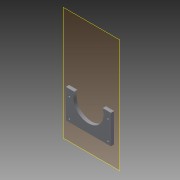
# Autodesk Inventor part: outputGearSupport
Saved by Autodesk Inventor 2013 (Build 170138000, 138)
## iProperties
Created: 2014-07-02
Part Number: outputGearSupport
Material: Generic
Document SubType Name: Modeling
Designer: Nano
Density: 1 g/cm^3
Author: Nano
Autodesk Inventor part; units mm, degrees
ref_plane "YZ Plane" through (0, 0, 0) normal (1, 0, 0) x (0, 1, 0)
ref_plane "XZ Plane" through (0, 0, 0) normal (0, 1, 0) x (-1, 0, 0)
ref_plane "XY Plane" through (0, 0, 0) normal (0, 0, 1) x (1, 0, 0)
ref_plane "Work Plane1" through (0, 0, 0) normal (0, 0, 1) x (1, 0, 0)
sketch "Sketch1" plane through (0, 0, 0) normal (0, 0, 1) x (1, 0, 0)
  circle A0 centre (0, -25.4) radius 24.765 construction
  arc A1 (-28.1777, -15.24) -> (28.1777, -15.24) centre (0, -25.4) ccw
  line L0 (-44.45, -72.39) -> (44.45, -72.39)
  line L1 (44.45, -72.39) -> (44.45, -15.24)
  line L2 (-44.45, -15.24) -> (-44.45, -72.39)
  line L3 (44.45, -15.24) -> (28.1777, -15.24)
  line L4 (-28.1777, -15.24) -> (-44.45, -15.24)
  point P0 (0, 0)
  dimension "d0" = 88.9
  dimension "d1" = 57.15
  dimension "d2" = 44.45
  dimension "d3" = 44.45
  dimension "d4" = 46.99
  dimension "d5" = 29.9535
  dimension "d6" = 88.9
  constraints: 10 end point, 3 parallel, 2 point on circle, 1 centre point, 1 horizontal, 1 perpendicular
  measures "d0" distance of L2.start L1.end
  measures "d1" distance of L1.end L0.end
  measures "d2" distance from line of L1 A0.centre
  measures "d3" distance from line of L2 A0.centre
  measures "d4" distance from line of L0 A0.centre
  measures "d5" radius of A1
  measures "d6" distance between parallel lines of L2 L1
extrude "Extrusion1" add sketch "Sketch1" along normal blind 6.35
sketch "Sketch2" plane through (0, 0, 6.35) normal (0, 0, 1) x (1, 0, 0)
  line L0 (-44.45, -72.39) -> (44.45, -72.39) projected
  line L1 (44.45, -72.39) -> (44.45, -15.24) projected
  line L2 (-44.45, -15.24) -> (-44.45, -72.39) projected
  circle A0 centre (-38.1, -66.04) radius 1.8542
  circle A1 centre (38.1, -66.04) radius 1.8542
  circle A2 centre (-38.1, -27.94) radius 1.8542
  circle A3 centre (38.1, -27.94) radius 1.8542
  point P0 (0, 0)
  dimension "d9" = 3.7084
  dimension "d10" = 3.7084
  dimension "d11" = 6.35
  dimension "d12" = 6.35
  dimension "d13" = 6.35
  dimension "d14" = 6.35
  dimension "d17" = 38.1
  constraints: 4 centre point, 1 vertical, 4 other
  measures "d9" diameter of A0
  measures "d10" diameter of A1
  measures "d11" distance from line of L2 A0.centre
  measures "d12" distance from line of L1 A1.centre
  measures "d13" distance from line of L0 A0.centre
  measures "d14" distance from line of L0 A1.centre
  measures "d17" distance of A0.centre A2.centre
extrude "Extrusion2" cut sketch "Sketch2" against normal through all
equation "\"d2\" = d3"
equation "\"d12\" = d11"
equation "\"d13\" = d11"
equation "\"d14\" = d11"
body "Solid1"
